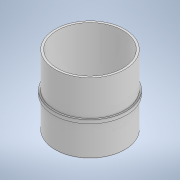
# Autodesk Inventor part: pld_bh
Saved by Autodesk Inventor 2022 (Build 260153000, 153)
## iProperties
Created: 2023-01-19
Part Number: pld_bh
Material: Generic
Document SubType Name: Modeling
Designer: Jasper
Density: 1 g/cm^3
Appearance: Default
Author: Jasper
Autodesk Inventor part; units mm, degrees
ref_plane "YZ Plane" through (0, 0, 0) normal (1, 0, 0) x (0, 1, 0)
ref_plane "XZ Plane" through (0, 0, 0) normal (0, 1, 0) x (-1, 0, 0)
ref_plane "XY Plane" through (0, 0, 0) normal (0, 0, 1) x (1, 0, 0)
sketch "Sketch1" plane through (0, 0, 0) normal (0, 0, 1) x (1, 0, 0)
  line L0 (0, 0) -> (0, 150)
  line L1 (46.5, 103.1016) -> (49.5, 103.1016)
  line L2 (49.5, 103.1016) -> (49.5, 4.6016)
  line L3 (48, 3.1016) -> (48, 3.1016)
  line L4 (46.5, 4.6016) -> (46.5, 103.1016)
  line L5 (49.5, 48.1016) -> (51.75, 48.1016)
  line L6 (51.75, 48.1016) -> (51.75, 53.1016)
  line L7 (51.75, 53.1016) -> (49.5, 53.1016)
  line L8 (49.5, 53.1016) -> (49.5, 48.1016)
  arc A0 (46.5, 4.6016) -> (48, 3.1016) centre (48, 4.6016) ccw
  arc A1 (48, 3.1016) -> (49.5, 4.6016) centre (48, 4.6016) ccw
  point P0 (49.5, 3.1016)
  point P1 (46.5, 3.1016)
  dimension "d1" = 100
  dimension "d2" = 50
  dimension "d3" = 5
  dimension "d4" = 3
  dimension "d5" = 99
  dimension "d6" = 103.5
  dimension "d8" = 1.5
  constraints: 18 end point, 5 point on line, 4 parallel, 4 point on circle, 4 tangent, 2 centre point, 2 horizontal, 2 perpendicular, 1 concentric, 1 vertical
  measures "d1" distance of point (46.5, 3.102) L1.start
  measures "d2" distance between parallel lines of L3 L7
  measures "d3" distance between parallel lines of L7 L5
  measures "d4" distance between parallel lines of L2 L4
  measures "d5" diameter of L2 L0
  measures "d6" diameter of L6 L0
  measures "d8" radius of A0
revolve "Revolution1" add sketch "Sketch1" angle 360 about axis through (0, 0, 0) along (0, 1, 0)
body "Solid1"
